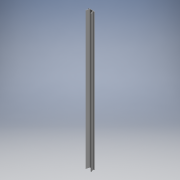
# Autodesk Inventor part: SLZ_63_Abdeck_Profil#_2871
Saved by Autodesk Inventor 2017.3 (Build 213256000, 256)
## iProperties
Part Number: SLZ_63_Abdeck_Profil#_2871
Material: Generic
Catalog Web Link: www.cadenas.de
Description: AbdeckProfil_SLZ63-Control-Tec
Vendor: ROSEKRIEGER
Document SubType Name: Modeling
Designer: partserver
Manufacturer: ROSEKRIEGER
Mass: 6.9387 g
Surface Area: 161.584 cm^2
Volume: 6.9387 cm^3
Density: 1 g/cm^3
Appearance: PSOLRGB-191-191-191
Category: PARTsolutions
Company: ROSEKRIEGER
Title: SLZ_63_Abdeck_Profil#_2871
Author: Cadenas PARTsolutions
Comments: Control-Tec
PSOL_IDENT_0: {$CADENAS_DATA\23d-libs\rose_krieger\linearkomponenten\pool_lineartechnik\_hubsaeule_zyliinder\elekt
PSOL_IDENT_1: rozylinder\elekzyl_slz63\parts\slz63_plfl_abdeck_profil.prj},205 {VTYP=3D},{NB=SLZ_63_Abdeck_Profil#
PSOL_IDENT_2: _2871},{LINA=SLZ_63_Abdeck_Profil#_2871},{NN=AbdeckProfil_SLZ63},{DATE=02.12.2020 11:16:22},{GEOMDAT
PSOL_IDENT_3: E=27.02.2017 15:55:00},{VERSION=},{LINEID=810},{WBVAR=},{WBNUMERIC=}  {NB=SLZ_63_Abdeck_Profil#_2871
PSOL_IDENT_4: },{LINA=SLZ_63_Abdeck_Profil#_2871},{KT=DUMMY},{IDNR=},{CODE=TQ3},{ARTIKEL=Elektrozylinder },{TYPE=S
PSOL_IDENT_5: LZ 63 Tr P PL},{BEST=SLZ_63_Abdeck_Profil},{VARIANTE=PL},{SPINDEL=Tr 28x10},{SPINDELCODE=1.000},{SCH
PSOL_IDENT_6: UTZARTVIS=IP54},{SCHUTZART=1},{HUB1=0,[0:200]},{HUB2=200},{L1=287},{HINWEINBAUX=Hub + 274,5 mm},{DUM
PSOL_IDENT_7: MYDURCH=10.000},{DUMMYLAENG=20.000},{HILFEHUB=105},{LAENDOPPROFIL=184.500},{RF=1.000},{GRUNDKOE=274.
PSOL_IDENT_8: 500},{A=100},{B=80},{C=100},{D=125},{E=238},{F=40},{G=M16x1.5},{H=104},{K=125},{L=105},{M=48},{N=56.
PSOL_IDENT_9: 5},{O=86},{P=18.5},{PPATH=sbl_lz70p_plfl.prj}
NB: SLZ_63_Abdeck_Profil#_2871
NN: AbdeckProfil_SLZ63
NT: Control-Tec
NBSYN: $BEST.#_$L1.$SCHUTZART.
LINA: SLZ_63_Abdeck_Profil#_2871
CATALOG: RK Rose+Krieger
ARTIKEL: Elektrozylinder
TYPE: SLZ 63 Tr P PL
BEST: SLZ_63_Abdeck_Profil
VARIANTE: PL
SPINDEL: Tr 28x10
SPINDELCODE: 1
SCHUTZARTVIS: IP54
SCHUTZART: 1
HUB1: 0,[0:200]
HUB2: 200
L1: 287
HINWEINBAUX: Hub + 274,5 mm
DUMMYDURCH: 10
DUMMYLAENG: 20
HILFEHUB: 105
LAENDOPPROFIL: 184.5
RF: 1
GRUNDKOE: 274.5
A: 100
B: 80
C: 100
D: 125
E: 238
F: 40
G: M16x1.5
H: 104
K: 125
L: 105
M: 48
N: 56.5
O: 86
P: 18.5
SUPPLIER: ROSEKRIEGER
ARTICLENO: SLZ_63_Abdeck_Profil#_2871
BOMINFO: SLZ_63_Abdeck_Profil#_2871
CREATOR: CADENAS GmbH
Autodesk Inventor part; units mm, degrees
sketch "Sketch_1" plane through (0, 0, 0) normal (0, 0, 1) x (1, 0, 0)
  line L0 (-6.5, -6.2) -> (-5, -7.8)
  line L1 (-5, -7.8) -> (-3.226, -1.1793)
  arc A0 (-3.0947, -1.0409) -> (-3.226, -1.1793) centre (-3.0328, -1.2311) ccw
  arc A1 (3.0947, -1.0409) -> (-3.0947, -1.0409) centre (0, -10.55) ccw
  arc A2 (3.226, -1.1793) -> (3.0947, -1.0409) centre (3.0328, -1.2311) ccw
  line L2 (3.226, -1.1793) -> (5, -7.8)
  line L3 (5, -7.8) -> (6.5, -6.2)
  line L4 (6.5, -6.2) -> (5.326, -5.9257)
  line L5 (5.326, -5.9257) -> (4.9136, -4.3864)
  line L6 (4.9136, -4.3864) -> (5.5, -3.8)
  line L7 (5.5, -3.8) -> (4.4843, -2.7843)
  line L8 (4.4843, -2.7843) -> (4.0598, -1.2)
  line L9 (4.0598, -1.2) -> (5.8, -1.2)
  arc A3 (5.8, -1.2) -> (6, -1) centre (5.8, -1) ccw
  line L10 (6, -1) -> (6, -0.2)
  arc A4 (6, -0.2) -> (5.8, 0) centre (5.8, -0.2) ccw
  line L11 (5.8, 0) -> (-5.8, 0)
  arc A5 (-5.8, 0) -> (-6, -0.2) centre (-5.8, -0.2) ccw
  line L12 (-6, -0.2) -> (-6, -1)
  arc A6 (-6, -1) -> (-5.8, -1.2) centre (-5.8, -1) ccw
  line L13 (-5.8, -1.2) -> (-4.0598, -1.2)
  line L14 (-4.0598, -1.2) -> (-4.4843, -2.7843)
  line L15 (-4.4843, -2.7843) -> (-5.5, -3.8)
  line L16 (-5.5, -3.8) -> (-4.9136, -4.3864)
  line L17 (-4.9136, -4.3864) -> (-5.326, -5.9257)
  line L18 (-5.326, -5.9257) -> (-6.5, -6.2)
  constraints: 38 end point, 14 point on circle, 7 centre point
extrude "Extrusion1" add sketch "Sketch_1" along normal blind 287
ref_plane "ABDECKPROFIL_XY" through (0, 0, 287) normal (0, 0, -1) x (1, 0, 0)
ref_plane "ABDECKPROFIL_YZ" through (0, 0, 287) normal (1, 0, 0) x (0, -1, 0)
ref_plane "ABDECKPROFIL_ZX" through (0, 0, 287) normal (0, -1, 0) x (0, 0, -1)
body "Solid1"
